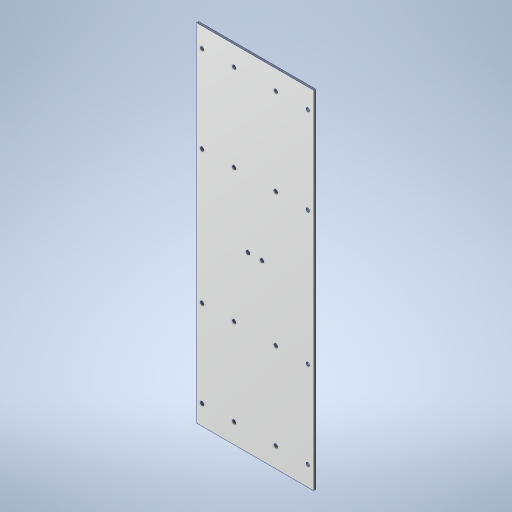
# Autodesk Inventor part: Rear Internal Side Panel
Saved by Autodesk Inventor 2024 (Build 280153000, 153)
## iProperties
Created: 2024-09-28
Part Number: Rear Internal Side Panel
Material: Generic
Document SubType Name: Modeling
Designer: Ishaan
Density: 1 g/cm^3
Appearance: Default
Author: Ishaan
Autodesk Inventor part; units mm, degrees
ref_plane "YZ Plane" through (0, 0, 0) normal (1, 0, 0) x (0, 1, 0)
ref_plane "XZ Plane" through (0, 0, 0) normal (0, 1, 0) x (-1, 0, 0)
ref_plane "XY Plane" through (0, 0, 0) normal (0, 0, 1) x (1, 0, 0)
sketch "Sketch1" plane through (0, 0, 0) normal (0, 0, 1) x (1, 0, 0)
  line L0 (84.75, -249.5) -> (-84.75, -249.5)
  line L1 (-84.75, -249.5) -> (-84.75, 249.5)
  line L2 (-84.75, 249.5) -> (84.75, 249.5)
  line L3 (84.75, 249.5) -> (84.75, -249.5)
  line L4 (84.75, -249.5) -> (-84.75, 249.5) construction
  line L5 (-84.75, -249.5) -> (84.75, 249.5) construction
  point P0 (0, 0)
  dimension "d0" = 169.5
  dimension "d1" = 499
  constraints: 12 end point, 2 midpoint, 2 parallel, 1 horizontal, 1 perpendicular
  measures "d0" distance of L1.end L2.end
  measures "d1" distance of L0.end L1.end
extrude "Extrusion1" add sketch "Sketch1" along normal mid plane 3
extrude "Extrusion2" cut sketch "Sketch1" along normal mid plane 2.9
extrude "Extrusion3" add sketch "Sketch1" along normal mid plane 2.9 separate body
sketch "Sketch4" plane through (0, 0, 1.5) normal (0, 0, 1) x (1, 0, 0)
  line L0 (30, -221) -> (-30, -221)
  line L1 (-30, -221) -> (-30, 221)
  line L2 (-30, 221) -> (30, 221)
  line L3 (30, 221) -> (30, -221)
  line L4 (30, -221) -> (-30, 221) construction
  line L5 (-30, -221) -> (30, 221) construction
  line L6 (30, -96) -> (-30, -96)
  line L7 (-30, -96) -> (-30, 96)
  line L8 (-30, 96) -> (30, 96)
  line L9 (30, 96) -> (30, -96)
  line L10 (30, -96) -> (-30, 96) construction
  line L11 (-30, -96) -> (30, 96) construction
  line L12 (-10, 0) -> (10, 0) construction
  point P0 (0, 0)
  dimension "d28" = 60
  dimension "d29" = 442
  dimension "d30" = 125
  dimension "d31" = 20
  constraints: 26 end point, 10 coincident, 5 midpoint, 4 parallel, 3 horizontal, 2 perpendicular, 1 point on line
  measures "d28" distance of L1.end L2.end
  measures "d29" distance of L0.end L1.end
  measures "d30" distance between parallel lines of L2 L8
  measures "d31" distance of L12.start L12.end
hole "Hole2" at (-30, 221, 1.5) at (30, 221, 1.5) at (-30, 96, 1.5) at (30, 96, 1.5) at (-30, -96, 1.5) at (30, -96, 1.5) at (30, -221, 1.5) at (-30, -221, 1.5) at (-10, 0, 1.5) at (10, 0, 1.5) direction (0, 0, -1) diameter 5.4 end through all bodies 1 2
sketch "Sketch5" plane through (0, 0, -1.5) normal (0, 0, -1) x (-1, 0, 0)
  line L0 (-76, -96) -> (76, -96) construction
  line L1 (76, -96) -> (76, 96) construction
  line L2 (76, 96) -> (-76, 96) construction
  line L3 (-76, 96) -> (-76, -96) construction
  line L4 (-76, -96) -> (76, 96) construction
  line L5 (76, -96) -> (-76, 96) construction
  line L6 (-76, -221) -> (76, -221) construction
  line L7 (76, -221) -> (76, 221) construction
  line L8 (76, 221) -> (-76, 221) construction
  line L9 (-76, 221) -> (-76, -221) construction
  line L10 (-76, -221) -> (76, 221) construction
  line L11 (76, -221) -> (-76, 221) construction
  circle A0 centre (30, 96) radius 2.7 projected
  circle A1 centre (30, 221) radius 2.7 projected
  point P0 (0, 0)
  dimension "d39" = 152
  constraints: 24 end point, 7 coincident, 4 midpoint, 4 parallel, 4 point on line, 2 horizontal, 2 perpendicular, 1 collinear
  measures "d39" distance of L1.end L2.end
hole "Hole3" at (-76, 221, -1.5) at (76, 221, -1.5) at (76, 96, -1.5) at (-76, 96, -1.5) at (-76, -96, -1.5) at (76, -96, -1.5) at (76, -221, -1.5) at (-76, -221, -1.5) direction (0, 0, 1) diameter 5.4 end through all bodies 1 2
sketch "Sketch2" plane through (0, 0, 1.5) normal (0, 0, 1) x (1, 0, 0)
  line L0 (-84.75, -249.5) -> (84.75, -249.5) projected
  line L1 (60, -115) -> (-60, -115) construction
  line L2 (-60, -115) -> (-60, 135) construction
  line L3 (-60, 135) -> (60, 135) construction
  line L4 (60, 135) -> (60, -115) construction
  line L5 (60, -115) -> (-60, 135) construction
  line L6 (-60, -115) -> (60, 135) construction
  point P0 (0, 0)
  point P1 (0, 10)
  point P2 (0, 135)
  point P3 (-60, 10)
  point P4 (60, 10)
  point P5 (0, -115)
  point P6 (60, 10)
  point P7 (0, 10)
  point P8 (-60, 10)
  dimension "d19" = 250
  dimension "d20" = 120
  dimension "d22" = 10
  constraints: 12 end point, 7 coincident, 6 midpoint, 2 parallel, 1 horizontal, 1 perpendicular, 1 vertical alignment
  measures "d19" distance of L1.end L2.end
  measures "d20" distance of L2.end L3.end
  measures "d22" distance of point (0, 10) point (0, 0)
sketch "Sketch3" plane through (0, 0, 1.5) normal (0, 0, 1) x (1, 0, 0)
  line L0 (-12, -249.5) -> (12, -249.5)
  line L1 (12, -249.5) -> (12, -246.875)
  line L2 (11, -245.875) -> (-11, -245.875)
  line L3 (-12, -246.875) -> (-12, -249.5)
  line L4 (-84.75, -249.5) -> (84.75, -249.5) projected
  arc A0 (-11, -245.875) -> (-12, -246.875) centre (-11, -246.875) ccw
  arc A1 (12, -246.875) -> (11, -245.875) centre (11, -246.875) ccw
  point P0 (0, 0)
  point P1 (12, -245.875)
  point P2 (-12, -245.875)
  point P3 (0, -249.5)
  dimension "d23" = 24
  dimension "d24" = 3.625
  dimension "d27" = 1
  constraints: 8 end point, 4 point on circle, 4 point on line, 4 tangent, 2 centre point, 2 midpoint, 2 parallel, 1 equal radius, 1 horizontal, 1 perpendicular
  measures "d23" distance of point (-12, -245.875) point (12, -245.875)
  measures "d24" distance of point (12, -245.875) L0.end
  measures "d27" radius of A0
